Autodesk Inventor part; units mm, degrees
(part 2 of 2)
sketch "Sketch15" plane through (0, 0, 2) normal (0, 0, 1) x (1, 0, 0)
  line L0 (-89.4111, -249.9594) -> (-89.4111, -109.9594) projected
  line L1 (-89.4111, -109.9594) -> (-33.4111, -109.9594)
  line L2 (-33.4111, -109.9594) -> (-33.4111, -179.9594)
  line L3 (-33.4111, -179.9594) -> (-89.4111, -179.9594)
  line L4 (-89.4111, -179.9594) -> (-89.4111, -109.9594)
  line L5 (-33.4111, -179.9594) -> (19.7389, -179.9594)
  line L6 (19.7389, -179.9594) -> (19.7389, -170.9494)
  line L7 (19.7389, -170.9494) -> (-33.4111, -170.9494)
  line L8 (-33.4111, -170.9494) -> (-33.4111, -179.9594)
  circle A0 centre (19.7389, -170.9494) radius 1.75
  circle A1 centre (19.7389, -188.9694) radius 1.75
  line L9 (-33.4111, -179.9594) -> (19.7389, -179.9594)
  line L10 (19.7389, -179.9594) -> (19.7389, -148.9094)
  line L11 (19.7389, -148.9094) -> (-33.4111, -148.9094)
  line L12 (-33.4111, -148.9094) -> (-33.4111, -179.9594)
  line L13 (-33.4111, -179.9594) -> (19.7389, -179.9594)
  line L14 (19.7389, -179.9594) -> (19.7389, -139.9094)
  line L15 (19.7389, -139.9094) -> (-33.4111, -139.9094)
  line L16 (-33.4111, -139.9094) -> (-33.4111, -179.9594)
  circle A2 centre (19.7389, -148.9094) radius 1.75
  circle A3 centre (19.7389, -139.9094) radius 1.75
  circle A4 centre (19.7389, -211.0094) radius 1.75
  circle A5 centre (19.7389, -220.0094) radius 1.75
  circle A6 centre (-86.5611, -170.9494) radius 1.75
  circle A7 centre (-86.5611, -188.9694) radius 1.75
  circle A8 centre (-86.5611, -148.9094) radius 1.75
  circle A9 centre (-86.5611, -139.9094) radius 1.75
  circle A10 centre (-86.5611, -211.0094) radius 1.75
  circle A11 centre (-86.5611, -220.0094) radius 1.75
  line L17 (-15.4111, -37.2123) -> (-18, -37.2123)
  line L18 (-18, -37.2123) -> (-18, -32.7277)
  line L19 (-18, -32.7277) -> (-15.4111, -32.7277)
  line L20 (-15.4111, -32.7277) -> (-15.4111, -37.2123)
  line L21 (-15.4111, -37.2123) -> (-18, -32.7277) construction
  line L22 (-18, -37.2123) -> (-15.4111, -32.7277) construction
  circle A12 centre (-18, -32.7277) radius 1.75
  circle A13 centre (-15.4111, -32.7277) radius 1.75
  circle A14 centre (-18, -37.2123) radius 1.75
  circle A15 centre (-15.4111, -37.2123) radius 1.75
  line L23 (-51.4111, -211.1394) -> (-15.4111, -211.1394)
  line L24 (-15.4111, -211.1394) -> (-15.4111, -148.7794)
  line L25 (-15.4111, -148.7794) -> (-51.4111, -148.7794)
  line L26 (-51.4111, -148.7794) -> (-51.4111, -211.1394)
  line L27 (-51.4111, -211.1394) -> (-15.4111, -148.7794) construction
  line L28 (-15.4111, -211.1394) -> (-51.4111, -148.7794) construction
  circle A16 centre (-15.4111, -148.7794) radius 1.75
  circle A17 centre (-51.4111, -148.7794) radius 1.75
  circle A18 centre (-15.4111, -211.1394) radius 1.75
  circle A19 centre (-51.4111, -211.1394) radius 1.75
  line L29 (-2.2311, -18) -> (-64.5911, 18) construction
  line L30 (-64.5911, -18) -> (-2.2311, 18) construction
  circle A20 centre (-64.5911, 18) radius 1.75
  circle A21 centre (-2.2311, 18) radius 1.75
  circle A22 centre (-64.5911, -18) radius 1.75
  circle A23 centre (-2.2311, -18) radius 1.75
  line L31 (-33.4111, -130.9594) -> (-33.4111, -179.9594)
  line L32 (-64.5911, -197.9594) -> (-2.2311, -197.9594)
  line L33 (-2.2311, -197.9594) -> (-2.2311, -161.9594)
  line L34 (-2.2311, -161.9594) -> (-64.5911, -161.9594)
  line L35 (-64.5911, -161.9594) -> (-64.5911, -197.9594)
  line L36 (-64.5911, -197.9594) -> (-2.2311, -161.9594) construction
  line L37 (-2.2311, -197.9594) -> (-64.5911, -161.9594) construction
  circle A24 centre (-2.2311, -161.9594) radius 1.75
  circle A25 centre (-64.5911, -161.9594) radius 1.75
  circle A26 centre (-2.2311, -197.9594) radius 1.75
  circle A27 centre (-64.5911, -197.9594) radius 1.75
  line L38 (-33.4111, -179.9594) -> (-6.4111, -179.9594)
  line L39 (-6.4111, -179.9594) -> (-6.4111, -152.9594)
  line L40 (-6.4111, -152.9594) -> (-33.4111, -152.9594)
  line L41 (-33.4111, -152.9594) -> (-33.4111, -179.9594)
  circle A28 centre (-6.4111, -152.9594) radius 1.75
  circle A29 centre (-6.4111, -206.9594) radius 1.75
  circle A30 centre (-60.4111, -152.9594) radius 1.75
  circle A31 centre (-60.4111, -206.9594) radius 1.75
  circle A32 centre (-33.4111, -179.9594) radius 25.4313
  line L42 (22.5889, -109.9594) -> (22.5889, -249.9594) projected
  line L43 (-89.4111, -109.9594) -> (22.5889, -109.9594)
  line L44 (22.5889, -109.9594) -> (22.5889, -117.4593)
  line L45 (22.5889, -117.4593) -> (-89.4111, -117.4593)
  line L46 (-89.4111, -117.4593) -> (-89.4111, -109.9594)
  line L47 (-33.4111, -179.9594) -> (-48.7911, -179.9594)
  line L48 (-48.7911, -179.9594) -> (-48.7911, -117.4593)
  line L49 (-48.7911, -117.4593) -> (-33.4111, -117.4593)
  line L50 (-33.4111, -117.4593) -> (-33.4111, -179.9594)
  circle A33 centre (-48.7911, -117.4593) radius 1.75
  circle A34 centre (-62.1611, -117.4593) radius 1.75
  circle A35 centre (-73.0143, -117.4593) radius 1.75
  circle A36 centre (-83.5099, -117.4593) radius 1.75
  circle A37 centre (-33.4111, -117.4593) radius 1.75
  circle A38 centre (-18.0311, -117.4593) radius 1.75
  circle A39 centre (-4.6611, -117.4593) radius 1.75
  circle A40 centre (6.1922, -117.4593) radius 1.75
  circle A41 centre (16.6877, -117.4593) radius 1.75
  circle A42 centre (-48.7911, -242.4595) radius 1.75
  circle A43 centre (-62.1611, -242.4595) radius 1.75
  circle A44 centre (-73.0143, -242.4595) radius 1.75
  circle A45 centre (-83.5099, -242.4595) radius 1.75
  circle A46 centre (-33.4111, -242.4595) radius 1.75
  circle A47 centre (16.6877, -242.4595) radius 1.75
  circle A48 centre (6.1922, -242.4595) radius 1.75
  circle A49 centre (-4.6611, -242.4595) radius 1.75
  circle A50 centre (-18.0311, -242.4595) radius 1.75
  line L51 (-68.8662, -129.0528) -> (6.1922, -129.0528)
  line L52 (6.1922, -129.0528) -> (6.1922, -133.0339)
  line L53 (6.1922, -133.0339) -> (-68.8662, -133.0339)
  line L54 (-68.8662, -133.0339) -> (-68.8662, -129.0528)
  line L55 (-68.8662, -139.9094) -> (6.1922, -139.9094)
  line L56 (6.1922, -139.9094) -> (6.1922, -143.6344)
  line L57 (6.1922, -143.6344) -> (-68.8662, -143.6344)
  line L58 (-68.8662, -143.6344) -> (-68.8662, -139.9094)
  line L59 (-68.8662, -230.8661) -> (6.1922, -230.8661)
  line L60 (6.1922, -230.8661) -> (6.1922, -226.885)
  line L61 (6.1922, -226.885) -> (-68.8662, -226.885)
  line L62 (-68.8662, -226.885) -> (-68.8662, -230.8661)
  line L63 (-68.8662, -220.0094) -> (6.1922, -220.0094)
  line L64 (6.1922, -220.0094) -> (6.1922, -216.2845)
  line L65 (6.1922, -216.2845) -> (-68.8662, -216.2845)
  line L66 (-68.8662, -216.2845) -> (-68.8662, -220.0094)
  point P0 (0, 0)
  point P1 (-16.7055, -34.97)
  point P2 (-33.4111, 0)
  dimension "d164" = 56
  dimension "d165" = 70
  dimension "d166" = 53.15
  dimension "d167" = 9.01
  dimension "d168" = 3.5
  dimension "d171" = 31.05
  dimension "d172" = 40.05
  dimension "d173" = 3.5
  dimension "d174" = 3.5
  dimension "d175" = 3.5
  dimension "d176" = 3.5
  dimension "d177" = 3.5
  dimension "d178" = 3.5
  dimension "d180" = 62.36
  dimension "d181" = 3.5
  dimension "d182" = 3.5
  dimension "d183" = 3.5
  dimension "d184" = 3.5
  dimension "d185" = 36
  dimension "d187" = 36
  dimension "d188" = 3.5
  dimension "d189" = 3.5
  dimension "d190" = 3.5
  dimension "d191" = 3.5
  dimension "d192" = 49
  dimension "d193" = 36
  dimension "d194" = 3.5
  dimension "d195" = 3.5
  dimension "d196" = 3.5
  dimension "d197" = 3.5
  dimension "d198" = 27
  dimension "d199" = 27
  dimension "d200" = 3.5
  dimension "d210" = 15.38
  dimension "d211" = 3.5
  dimension "d212" = 3.5
  dimension "d213" = 3.5
  dimension "d214" = 3.5
  dimension "d215" = 3.5
  constraints: 130 end point, 51 centre point, 33 symmetric about line, 24 parallel, 23 coincident, 12 horizontal, 12 perpendicular, 10 point on line, 8 midpoint, 1 vertical, 25 other
  measures "d164" distance of L2.end L3.end
  measures "d165" distance of L1.end L2.end
  measures "d166" distance of L7.end L6.end
  measures "d167" distance of L5.end L6.end
  measures "d168" diameter of A0
  measures "d171" distance of L9.end L10.end
  measures "d172" distance of L13.end L14.end
  measures "d173" diameter of A2
  measures "d174" diameter of A3
  measures "d175" diameter of A12
  measures "d176" diameter of A13
  measures "d177" diameter of A14
  measures "d178" diameter of A15
  measures "d180" distance of L25.end L23.start
  measures "d181" diameter of A16
  measures "d182" diameter of A17
  measures "d183" diameter of A18
  measures "d184" diameter of A19
  measures "d185" distance of L23.start L23.end
  measures "d187" distance of L30.start L29.end
  measures "d188" diameter of A20
  measures "d189" diameter of A21
  measures "d190" diameter of A22
  measures "d191" diameter of A23
  measures "d192" distance of L2.end L31.start
  measures "d193" distance of L32.end L33.end
  measures "d194" diameter of A24
  measures "d195" diameter of A25
  measures "d196" diameter of A26
  measures "d197" diameter of A27
  measures "d198" distance of L39.end L40.end
  measures "d199" distance of L38.end L39.end
  measures "d200" diameter of A28
  measures "d210" distance of L48.end L49.end
  measures "d211" diameter of A33
  measures "d212" diameter of A34
  measures "d213" diameter of A35
  measures "d214" diameter of A36
  measures "d215" diameter of A37
extrude "Extrusion11" cut sketch "Sketch15" against normal blind 2 contours A36 L45 | L45 A36 | A32 L26 L3 | L3 L26 A32 | A25 L34 L35 | L35 L34 A25 | A27 L32 L35 | L35 L32 A27 | L26 A32 L34 L48 L3 | L3 L5 L24 A32 L32 L26 | A37 L45 L2 | L2 L45 A37 | A35 L45 | L45 A35 | L48 L34 L2 L3 | A32 L48 L34 | L32 A32 | L45 A37 L2 | L2 A37 L45 | L2 L7 L24 L5 | L48 A32 L2 L34 | A17 L25 L26 | L26 L25 A17 | A19 L23 L26 | L26 L23 A19 | A38 L45 | L45 A38 | A33 L48 L45 | L45 A33 | A41 L45 | L45 A41 | A34 L45 | L45 A34 | L2 L34 A32 L24 L7 | L24 L7 A32 L5 | L5 A32 L24 | L2 A32 L34 | L51 L52 L53 L2 | L2 L53 L48 L51 | L48 A33 L45 | L24 A32 L7 | L57 L58 L55 L48 | L48 L55 L2 L57 | A18 L24 L23 | L23 L24 A18 | A26 L33 L32 | L32 L33 A26 | L48 L53 L54 L51 | A39 L45 | L45 A39 | A40 L45 | L45 A40 | L2 L15 L56 L57 | A16 L11 L24 L25 | L25 L24 L11 A16 | L11 L24 A16 | L24 L11 A16 | A28 L39 L40 | L40 L39 A28 | A24 L33 L34 | L34 L33 A24 | A0 L10 L7 | L7 L6 A0 | L6 L10 A0 | A2 L14 L11 | L11 L10 A2 | A3 L14 L15 | L15 L14 A3 | L14 A2 L10 | A1 | A4 | A5 | A6 | A7 | A8 | A9 | A10 | A11 | A29 | A30 | A31 | A42 | A43 | A44 | A45 | A46 | A47 | A48 | A49 | A50 | L62 L61 L60 L59 | L66 L65 L64 L63
fillet "Fillet6" radius 1 16 edges at (-68.8662, -133.0339, 1) (-68.8662, -129.0528, 1) (6.1922, -129.0528, 1) (6.1922, -133.0339, 1) (-68.8662, -139.9094, 1) (-68.8662, -143.6344, 1) (6.1922, -143.6344, 1) (6.1922, -139.9094, 1) (6.1922, -230.8661, 1) (-68.8662, -226.885, 1) (-68.8662, -230.8661, 1) (-68.8662, -220.0094, 1) (-68.8662, -216.2845, 1) (6.1922, -220.0094, 1) (6.1922, -216.2845, 1) (6.1922, -226.885, 1)
sketch "Sketch17" plane through (0, 0, 2) normal (0, 0, 1) x (1, 0, 0)
  line L0 (22.5889, -109.9594) -> (22.5889, -249.9594) projected
  line L1 (25, -110) -> (25, -138.8544) projected
  line L2 (22.5889, -116.5482) -> (25, -116.5482)
  line L3 (25, -116.5482) -> (25, -117.4993)
  line L4 (25, -117.4993) -> (22.5889, -117.4993)
  line L5 (22.5889, -117.4993) -> (22.5889, -116.5482)
  line L6 (22.5889, -130.5648) -> (25, -130.5648)
  line L7 (25, -130.5648) -> (25, -131.6661)
  line L8 (25, -131.6661) -> (22.5889, -131.6661)
  line L9 (22.5889, -131.6661) -> (22.5889, -130.5648)
  line L10 (25, -212) -> (25, -238) projected
  line L11 (22.5889, -227.9951) -> (25, -227.9951)
  line L12 (25, -227.9951) -> (25, -228.8643)
  line L13 (25, -228.8643) -> (22.5889, -228.8643)
  line L14 (22.5889, -228.8643) -> (22.5889, -227.9951)
  line L15 (23, -108) -> (9.255, -108) projected
  line L16 (-89.4111, -109.9594) -> (22.5889, -109.9594) projected
  line L17 (12.9091, -108) -> (14.007, -108)
  line L18 (14.007, -108) -> (14.007, -109.9594)
  line L19 (14.007, -109.9594) -> (12.9091, -109.9594)
  line L20 (12.9091, -109.9594) -> (12.9091, -108)
  line L21 (107.4375, -108.4648) -> (58.6375, -108.4648) projected
  line L22 (53.325, -111) -> (112.325, -111) projected
  line L23 (80.7979, -108.4648) -> (81.8044, -108.4648)
  line L24 (81.8044, -108.4648) -> (81.8044, -111)
  line L25 (81.8044, -111) -> (80.7979, -111)
  line L26 (80.7979, -111) -> (80.7979, -108.4648)
  point P0 (0, 0)
  constraints: 40 end point, 10 parallel, 10 point on line, 5 horizontal, 5 perpendicular
extrude "Extrusion12" add sketch "Sketch17" against normal blind 2 contours L11 L10 L13 L0 | L2 L1 L4 L0 | L16 L20 L15 L18 | L6 L1 L8 L0 | L24 L22 L26 L21
body "Solid1"
